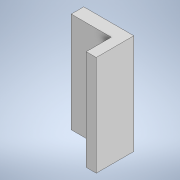
# Autodesk Inventor part: diffuser holder
Saved by Autodesk Inventor 2022.1 (Build 261234000, 234)
## iProperties
Created: 2022-02-25
Part Number: diffuser holder
Material: Generic
Document SubType Name: Modeling
Designer: Alif
Density: 1 g/cm^3
Appearance: Default
Author: Alif
Autodesk Inventor part; units mm, degrees
ref_plane "YZ Plane" through (0, 0, 0) normal (1, 0, 0) x (0, 1, 0)
ref_plane "XZ Plane" through (0, 0, 0) normal (0, 1, 0) x (-1, 0, 0)
ref_plane "XY Plane" through (0, 0, 0) normal (0, 0, 1) x (1, 0, 0)
sketch "Sketch1" plane through (0, 0, 0) normal (0, 0, 1) x (1, 0, 0)
  line L0 (0, 2.4078) -> (0, -18.8352)
  line L1 (-12.7, 4.1621) -> (-12.7, -19.6361)
  line L2 (-20.3324, 0) -> (-11.9249, 0)
  circle A0 centre (-12.7, 12.7) radius 3.175
  circle A1 centre (-12.7, -12.7) radius 3.175
  line L3 (-26.1938, 25.4) -> (-0.7938, 25.4)
  line L4 (-0.7938, 25.4) -> (-0.7937, -25.4)
  line L5 (-0.7937, -25.4) -> (-26.1937, -25.4)
  line L6 (-26.1937, -25.4) -> (-26.1938, 25.4)
  point P0 (0, 0)
  dimension "d0" = 12.7
  dimension "d1" = 25.4
  dimension "d2" = 25.4
  dimension "d3" = 6.35
  dimension "d4" = 6.35
  dimension "d5" = 1.5875
  dimension "d6" = 25.4
  dimension "d7" = 50.8
  dimension "d8" = 12.7
  constraints: 14 end point, 2 centre point, 2 horizontal, 2 parallel, 2 point on line, 2 vertical, 1 perpendicular
  measures "d0" distance between parallel lines of L0 L1
  measures "d1" diameter of A0.centre L2
  measures "d2" diameter of A1.centre L2
  measures "d3" diameter of A0
  measures "d4" diameter of A1
  measures "d5" diameter of L4 L0
  measures "d6" distance of L3.start L3.end
  measures "d7" distance of L5.end L3.start
  measures "d8" distance from line of A0.centre L3
extrude "Extrusion1" add sketch "Sketch1" along normal blind 6.35
sketch "Sketch2" plane through (0, 0, 6.35) normal (0, 0, 1) x (1, 0, 0)
  line L0 (-0.7938, 25.4) -> (-26.1938, 25.4) projected
  line L1 (-0.7937, -25.4) -> (-0.7938, 25.4) projected
  line L2 (-5.8738, 25.4) -> (-0.7937, 25.4)
  line L3 (-0.7937, 25.4) -> (-0.7937, -25.4)
  line L4 (-0.7937, -25.4) -> (-5.8737, -25.4)
  line L5 (-5.8737, -25.4) -> (-5.8738, 25.4)
  point P0 (0, 0)
  dimension "d11" = 5.08
  constraints: 8 end point, 2 parallel, 1 horizontal, 1 perpendicular, 1 point on line
  measures "d11" distance between parallel lines of L5 L1
extrude "Extrusion2" add sketch "Sketch2" along normal blind 12.7
body "Solid1"
